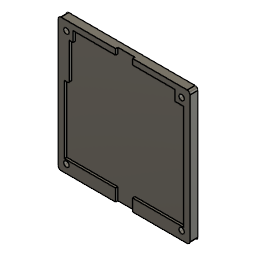
pin_grid_wafer_jig_al (Autodesk Fusion 360 design; units mm, degrees)
part number: 2026-08-14-01-45-42-701
Autodesk Fusion 360 part; units mm, degrees
ref_plane "WorkPlane1" through (0, 0, 7) normal (0, 0, 1) x (1, 0, 0)
sketch "Base Plate Sketch" plane through (0, 0, 0) normal (0, 0, 1) x (1, 0, 0)
  line L0 (-58.1813, -58.1813) -> (58.1813, -58.1813)
  line L1 (58.1813, -58.1813) -> (58.1813, 59)
  line L2 (58.1813, 59) -> (-58.1813, 59)
  line L3 (-58.1813, 59) -> (-58.1813, -58.1813)
extrude "Base Plate" add sketch "Base Plate Sketch" along normal blind 7
fillet "Fillet1" radius 2.5 4 edges at (-58.1813, 59, 3.5) (58.1813, 59, 3.5) (58.1813, -58.1813, 3.5) (-58.1813, -58.1813, 3.5)
sketch "Wafer Nest Pocket Sketch" plane through (0, 0, 7) normal (0, 0, 1) x (1, 0, 0)
  line L0 (-52.5, -47.4607) -> (52.5, -47.4607)
  line L1 (52.5, -47.4607) -> (52.5, 54)
  line L2 (52.5, 54) -> (-52.5, 54)
  line L3 (-52.5, 54) -> (-52.5, -47.4607)
extrude "Wafer Nest Pocket" cut sketch "Wafer Nest Pocket Sketch" against normal blind 2
sketch "Front-Center Access Relief Sketch" plane through (0, 0, 7) normal (0, 0, 1) x (1, 0, 0)
  line L0 (-7.5, -59.1812) -> (7.5, -59.1812)
  line L1 (7.5, -59.1812) -> (7.5, -44.4607)
  line L2 (7.5, -44.4607) -> (-7.5, -44.4607)
  line L3 (-7.5, -44.4607) -> (-7.5, -59.1812)
extrude "Front-Center Access Relief" cut sketch "Front-Center Access Relief Sketch" against normal blind 2
sketch "Rear-Center Access Relief Sketch" plane through (0, 0, 7) normal (0, 0, 1) x (1, 0, 0)
  line L0 (-7.5, 51) -> (7.5, 51)
  line L1 (7.5, 51) -> (7.5, 60)
  line L2 (7.5, 60) -> (-7.5, 60)
  line L3 (-7.5, 60) -> (-7.5, 51)
extrude "Rear-Center Access Relief" cut sketch "Rear-Center Access Relief Sketch" against normal blind 2
sketch "X Datum Square Sketch (165 deg / 9:30)" plane through (0, 0, 7) normal (0, 0, 1) x (1, 0, 0)
  line L0 (-56.2622, 20.1998) -> (-48.2622, 20.1998)
  line L1 (-48.2622, 20.1998) -> (-48.2622, 13.1998)
  arc A0 (-49.2622, 12.1998) -> (-48.2622, 13.1998) centre (-49.2622, 13.1998) ccw
  line L2 (-49.2622, 12.1998) -> (-56.2622, 12.1998)
  line L3 (-56.2622, 12.1998) -> (-56.2622, 20.1998)
extrude "X Datum Square (165 deg / 9:30, rounded corner)" add sketch "X Datum Square Sketch (165 deg / 9:30)" against normal blind 2
sketch "Left Wall Flush Above X-Datum Sketch" plane through (0, 0, 7) normal (0, 0, 1) x (1, 0, 0)
  line L0 (-52.5, 20.1998) -> (-48.2622, 20.1998)
  line L1 (-48.2622, 20.1998) -> (-48.2622, 54)
  line L2 (-48.2622, 54) -> (-52.5, 54)
  line L3 (-52.5, 54) -> (-52.5, 20.1998)
extrude "Left Wall Flush Above X-Datum" add sketch "Left Wall Flush Above X-Datum Sketch" against normal blind 2
sketch "Corner Clip (dowel -50.8, +50.8) Sketch" plane through (0, 0, 7) normal (0, 0, 1) x (1, 0, 0)
  line L0 (-52.5, 44.9187) -> (-44.9187, 44.9187)
  line L1 (-44.9187, 44.9187) -> (-44.9187, 54)
  line L2 (-44.9187, 54) -> (-52.5, 54)
  line L3 (-52.5, 54) -> (-52.5, 44.9187)
extrude "Corner Clip (dowel -50.8, +50.8)" add sketch "Corner Clip (dowel -50.8, +50.8) Sketch" against normal blind 2
sketch "Corner Clip (dowel +50.8, +50.8) Sketch" plane through (0, 0, 7) normal (0, 0, 1) x (1, 0, 0)
  line L0 (44.9187, 44.9187) -> (52.5, 44.9187)
  line L1 (52.5, 44.9187) -> (52.5, 54)
  line L2 (52.5, 54) -> (44.9187, 54)
  line L3 (44.9187, 54) -> (44.9187, 44.9187)
extrude "Corner Clip (dowel +50.8, +50.8)" add sketch "Corner Clip (dowel +50.8, +50.8) Sketch" against normal blind 2
sketch "Outer Front Left Dowel Bore Sketch" plane through (0, 0, 7) normal (0, 0, 1) x (1, 0, 0)
  circle A0 centre (-50.8, -50.8) radius 2.3813
extrude "Outer Front Left Dowel Bore" cut sketch "Outer Front Left Dowel Bore Sketch" against normal blind 7
sketch "Outer Front Right Dowel Bore Sketch" plane through (0, 0, 7) normal (0, 0, 1) x (1, 0, 0)
  circle A0 centre (50.8, -50.8) radius 2.3813
extrude "Outer Front Right Dowel Bore" cut sketch "Outer Front Right Dowel Bore Sketch" against normal blind 7
sketch "Outer Rear Left Dowel Bore Sketch" plane through (0, 0, 7) normal (0, 0, 1) x (1, 0, 0)
  circle A0 centre (-50.8, 50.8) radius 2.3813
extrude "Outer Rear Left Dowel Bore" cut sketch "Outer Rear Left Dowel Bore Sketch" against normal blind 7
sketch "Outer Rear Right Dowel Bore Sketch" plane through (0, 0, 7) normal (0, 0, 1) x (1, 0, 0)
  circle A0 centre (50.8, 50.8) radius 2.3813
extrude "Outer Rear Right Dowel Bore" cut sketch "Outer Rear Right Dowel Bore Sketch" against normal blind 7
equation "gridPitch = 25.4 mm" comment "Table hole-grid pitch"
equation "indexMove = 50.8 mm" comment "Two-grid-space indexing move"
equation "outerPinPatternSpan = 101.6 mm" comment "Four-space outer pin span"
equation "dowelDiameter = 4.7625 mm" comment "3/16 in steel locating dowel diameter"
equation "dowelHoleDiameter = 4.7625 mm" comment "3/16 in reamed dowel bore"
equation "plateEdgeMargin = 5.0 mm" comment "Solid margin, plate edge to nearest feature"
equation "plateWidth = 116.3625 mm" comment "Computed plate width (X)"
equation "plateHeight = 117.18125 mm" comment "Computed plate height (Y)"
equation "baseThickness = 7.0 mm" comment "Base plate thickness"
equation "pocketDepth = 2.0 mm" comment "Wafer-nest pocket depth"
equation "nestClearanceSide = 2.5 mm" comment "Left/right pocket-wall clearance"
equation "nestClearanceRear = 4.0 mm" comment "Rear pocket-wall clearance"
equation "filletRadius = 2.5 mm" comment "Base-plate corner fillet radius"
equation "primaryFlatClearance = 0.175 mm" comment "Front wall forward of nominal flat"
equation "xDatumSize = 8.0 mm" comment "Square X-datum block side"
equation "nestReliefWidth = 15.0 mm" comment "Front/rear access relief width"
equation "nestOffsetX = 0.0 mm" comment "Nest X from pin-square center"
equation "nestOffsetY = 0.0 mm" comment "Nest Y from pin-square center"
